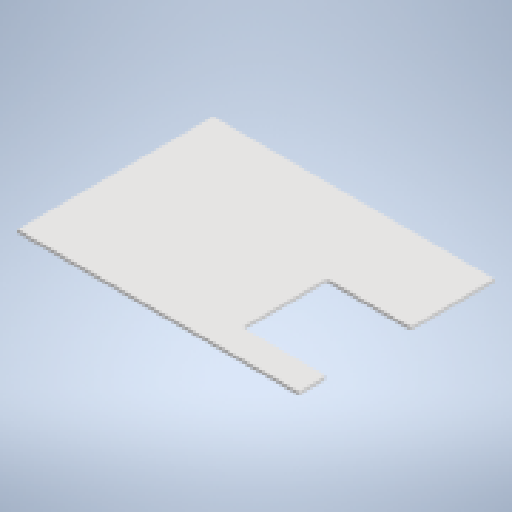
# Autodesk Inventor part: Grundplatte
Saved by Autodesk Inventor 2023 (Build 270158000, 158)
## iProperties
Created: 2023-11-24
Part Number: Grundplatte
Material: Generic
Document SubType Name: Modeling
Designer: danie
Density: 1 g/cm^3
Appearance: Default
Author: danie
Autodesk Inventor part; units mm, degrees
ref_plane "YZ Plane" through (0, 0, 0) normal (1, 0, 0) x (0, 1, 0)
ref_plane "XZ Plane" through (0, 0, 0) normal (0, 1, 0) x (-1, 0, 0)
ref_plane "XY Plane" through (0, 0, 0) normal (0, 0, 1) x (1, 0, 0)
sketch "Sketch1" plane through (0, 0, 0) normal (0, 1, 0) x (-1, 0, 0)
  line L0 (555, 500) -> (-555, 500)
  line L1 (-555, 500) -> (-555, -500)
  line L2 (-555, -500) -> (555, -500)
  line L3 (555, -500) -> (555, 500)
  line L4 (555, 500) -> (-555, -500) construction
  line L5 (-555, 500) -> (555, -500) construction
  line L6 (235, 50) -> (505, 50)
  line L7 (505, 50) -> (505, 450)
  line L8 (505, 450) -> (235, 450)
  line L9 (235, 450) -> (235, 50)
  line L10 (-135, 50) -> (135, 50)
  line L11 (135, 50) -> (135, 450)
  line L12 (135, 450) -> (-135, 450)
  line L13 (-135, 450) -> (-135, 50)
  line L14 (-505, 50) -> (-235, 50)
  line L15 (-235, 50) -> (-235, 450)
  line L16 (-235, 450) -> (-505, 450)
  line L17 (-505, 450) -> (-505, 50)
  line L18 (235, -450) -> (505, -450)
  line L19 (505, -450) -> (505, -50)
  line L20 (505, -50) -> (235, -50)
  line L21 (235, -50) -> (235, -450)
  line L22 (-135, -450) -> (135, -450)
  line L23 (135, -450) -> (135, -50)
  line L24 (135, -50) -> (-135, -50)
  line L25 (-135, -50) -> (-135, -450)
  line L26 (-505, -450) -> (-235, -450)
  line L27 (-235, -450) -> (-235, -50)
  line L28 (-235, -50) -> (-505, -50)
  line L29 (-505, -50) -> (-505, -450)
  line L30 (-555, 500) -> (-1155, 500)
  line L31 (-1155, 500) -> (-1155, -500)
  line L32 (-1155, -500) -> (-555, -500)
  line L33 (-555, -500) -> (-555, 500)
  line L34 (-555, 500) -> (-1155, 500)
  line L35 (-1155, 500) -> (-1155, 450)
  line L36 (-1155, 450) -> (-555, 450)
  line L37 (-555, 450) -> (-555, 500)
  line L38 (-555, -500) -> (-1155, -500)
  line L39 (-1155, -500) -> (-1155, -450)
  line L40 (-1155, -450) -> (-555, -450)
  line L41 (-555, -450) -> (-555, -500)
  line L42 (-1155, -500) -> (555, -500)
  line L43 (555, -500) -> (555, -550)
  line L44 (555, -550) -> (-1155, -550)
  line L45 (-1155, -550) -> (-1155, -500)
  line L46 (-1155, 500) -> (555, 500)
  line L47 (555, 500) -> (555, 550)
  line L48 (555, 550) -> (-1155, 550)
  line L49 (-1155, 550) -> (-1155, 500)
  line L50 (-555, 450) -> (-1155, 450)
  line L51 (-1155, 450) -> (-1155, -150)
  line L52 (-1155, -150) -> (-555, -150)
  line L53 (-555, -150) -> (-555, 450)
  point P0 (0, 0)
  point P1 (555, -525)
  dimension "d0" = 1000
  dimension "d1" = 1110
  dimension "d2" = 400
  dimension "d3" = 270
  dimension "d4" = 50
  dimension "d5" = 50
  dimension "d8" = 370
  dimension "d11" = 500
  dimension "d14" = 600
  dimension "d15" = 50
  dimension "d16" = 50
  dimension "d17" = 50
  dimension "d18" = 50
  dimension "d19" = 600
  dimension "d26" = 0
  dimension "d27" = 0
  constraints: 108 end point, 16 parallel, 9 horizontal, 8 perpendicular, 4 point on line, 3 midpoint, 1 vertical, 40 other
  measures "d0" distance of L2.end L0.start
  measures "d1" distance of L0.start L0.end
  measures "d2" distance of L6.end L7.end
  measures "d3" distance of L7.end L8.end
  measures "d4" distance between parallel lines of L3 L7
  measures "d5" distance between parallel lines of L0 L8
  measures "d8" distance of L6.start L10.start
  measures "d11" distance of L6.start L18.start
  measures "d14" distance of L32.end L31.end
  measures "d15" distance of L35.end L34.end
  measures "d16" distance of L38.end L39.end
  measures "d17" distance of L42.end L43.end
  measures "d18" distance of L47.end L46.end
  measures "d19" distance of L51.end L50.end
  measures "d26" distance between parallel lines of L2 L42
  measures "d27" distance from line of L3 point (555, -525)
extrude "Extrusion1" add sketch "Sketch1" along normal blind 25 contours L3 L2 L1 L0 | L0 L30 L49 L48 L47 | L1 L36 L31 L30 | L43 L44 L45 L32 L2 | L32 L31 L40 L1 | L1 L40 L31 L52 | L9 L8 L7 L6 | L13 L12 L11 L10 | L17 L16 L15 L14 | L21 L20 L19 L18 | L25 L24 L23 L22 | L29 L28 L27 L26
fillet "Fillet1" radius 20 4 edges at (555, 12.5, -150) (555, 12.5, 450) (1155, 12.5, 450) (1155, 12.5, -150)
chamfer "Chamfer1" distance 2 angle 45 20 edges at (855, 0, -150) (1149.1421, 0, -155.8579) (1155, 0, -335) (555, 0, 150) (855, 0, 450) (1149.1421, 0, 455.8579) (1155, 0, 485) (300, 0, 550) (-555, 0, 0) (300, 0, -550) (1155, 25, -335) (1149.1421, 25, -155.8579) (855, 25, -150) (555, 25, 150) (855, 25, 450) (1149.1421, 25, 455.8579) (1155, 25, 485) (300, 25, 550) (-555, 25, 0) (300, 25, -550)
equation "\"d0\" = Grundplatte_Width"
equation "\"d1\" = Grundplatte_Hight"
equation "\"d2\" = Palette_Width"
equation "\"d3\" = Palette_Hight"
equation "\"d4\" = Palette_Padding_Outer"
equation "\"d5\" = Palette_Padding_Outer"
equation "\"d8\" = Palette_Padding_Inner_X"
equation "\"d11\" = Palette_Padding_Inner_Y"
equation "\"d15\" = Palette_Padding_Outer"
equation "\"d16\" = Palette_Padding_Outer"
equation "\"d17\" = Palette_Padding_Outer"
equation "\"d18\" = Palette_Padding_Outer"
equation "\"Palette_Width\" = 400"
equation "\"Palette_Hight\" = 270"
equation "\"Palette_Padding_Outer\" = 0.5 * Palette_Padding"
equation "\"Palette_Padding_Inner_X\" = Palette_Hight + Palette_Padding"
equation "\"Palette_Padding_Inner_Y\" = Palette_Width + Palette_Padding"
equation "\"Grundplatte_Width\" = 1000"
equation "\"Grundplatte_Hight\" = 1110"
equation "\"Palette_Padding\" = 100"
body "Solid1"
